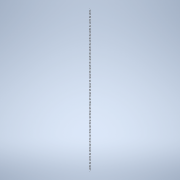
# Autodesk Inventor part: 10ft chain
Saved by Autodesk Inventor 2021 (Build 250183000, 183)
## iProperties
Created: 2021-02-06
Part Number: 10ft chain
Material: Generic
Document SubType Name: Modeling
Designer: aidan
Density: 1 g/cm^3
Appearance: Default
Author: aidan
Autodesk Inventor part; units mm, degrees
ref_plane "YZ Plane" through (0, 0, 0) normal (1, 0, 0) x (0, 1, 0)
sketch "Sketch1" plane through (0, 0, 0) normal (0, 0, 1) x (1, 0, 0)
  line L0 (0, -12.7) -> (0, 12.7)
  line L1 (9.525, -12.7) -> (9.525, 12.7)
  line L2 (-9.525, 12.7) -> (-9.525, -12.7)
  arc A0 (-9.525, -12.7) -> (9.525, -12.7) centre (0, -12.7) ccw
  arc A1 (9.525, 12.7) -> (-9.525, 12.7) centre (0, 12.7) ccw
  point P0 (0, 0)
  dimension "d1" = 9.525
  dimension "d2" = 25.4
  constraints: 8 end point, 4 point on circle, 4 tangent, 2 centre point, 1 midpoint, 1 parallel, 1 vertical
  measures "d1" radius of A1
  measures "d2" distance of L0.start L0.end
ref_plane "Work Plane1" through (9.525, 12.7, 0) normal (0, 1, 0) x (-1, 0, 0)
sketch "Sketch2" plane through (9.525, 12.7, 0) normal (0, 1, 0) x (-1, 0, 0)
  circle A0 centre (0, 0) radius 1.905
  point P0 (9.525, 0)
  point P1 (0, 0)
  dimension "d3" = 3.81
  constraints: 1 centre point, 1 coincident
  measures "d3" diameter of A0
sweep "Sweep1" add profiles "Sketch2" path "Sketch1" path curves L1 A0 L2 A1
sketch "Sketch3" plane through (0, 0, 0) normal (1, 0, 0) x (0, 1, 0)
  line L0 (-38.1, -9.525) -> (-12.7, -9.525)
  line L1 (-12.7, 9.525) -> (-38.1, 9.525)
  arc A0 (-38.1, 9.525) -> (-38.1, -9.525) centre (-38.1, 0) ccw
  arc A1 (-12.7, -9.525) -> (-12.7, 9.525) centre (-12.7, 0) ccw
  line L2 (-12.7, 1.905) -> (-12.7, -1.905) projected
  point P0 (0, 0)
  point P1 (0, 0)
  dimension "d6" = 9.525
  dimension "d7" = 25.4
  constraints: 4 end point, 4 point on circle, 4 tangent, 2 centre point, 1 coincident, 1 horizontal, 1 midpoint, 1 parallel
  measures "d6" radius of A1
  measures "d7" distance of A0.centre A1.centre
ref_plane "Work Plane2" through (0, -12.7, 0) normal (0, 1, 0) x (-1, 0, 0)
sketch "Sketch4" plane through (0, -12.7, 0) normal (0, 1, 0) x (-1, 0, 0)
  circle A0 centre (0, 9.525) radius 1.905
  point P0 (0, 0)
  point P1 (9.525, 0)
  point P2 (0, 0)
  point P3 (0, 0)
  point P4 (0, 0)
  point P5 (0, 9.525)
  dimension "d10" = 3.81
  constraints: 1 centre point, 1 coincident
  measures "d10" diameter of A0
sweep "Sweep2" add profiles "Sketch4" path "Sketch3" path curves L1 A0 L0 A1
pattern_linear "Rectangular Pattern1" count 72 spacing 50.8 along (0, -1, 0) of "Sweep2", "Sweep1"
body "Solid1"
